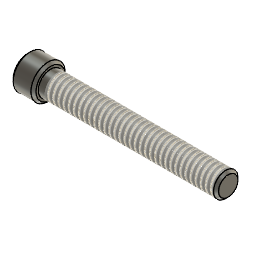
m2 bolt 6mm v2 (Autodesk Fusion 360 design; units mm, degrees)
Autodesk Fusion 360 part; units mm, degrees
sketch "Sketch1" plane through (0, 0, 0) normal (1, 0, 0) x (0, 1, 0)
  circle A0 centre (0, 0) radius 1.35
  line L0 (0, 0.866) -> (-0.75, 0.433)
  line L1 (-0.75, 0.433) -> (-0.75, -0.433)
  line L2 (-0.75, -0.433) -> (0, -0.866)
  line L3 (0, -0.866) -> (0.75, -0.433)
  line L4 (0.75, -0.433) -> (0.75, 0.433)
  line L5 (0.75, 0.433) -> (0, 0.866)
  line L6 (-0.75, -0.433) -> (0.75, 0.433) construction
  line L7 (0.75, -0.433) -> (-0.75, 0.433) construction
  line L8 (0, 0.866) -> (0, -0.866) construction
  line L9 (-0.75, -0.433) -> (0.75, -0.433) construction
  dimension "d1" = 1.5
  dimension "d2" = 2.7
  constraint coincident A0.centre origin
  constraint vertical L1
  constraint parallel L1 L4
  constraint equal L1 L2
  constraint equal L0 L1
  constraint equal L0 L5
  constraint equal L4 L5
  constraint equal L3 L4
  constraint midpoint L7 A0.centre
  constraint equal L6 L7
  constraint equal L7 L8
  measures "d1" distance of L1.end L3.end
  measures "d2" diameter of A0
extrude "Extrude1" add sketch "Sketch1" along normal blind 1.8 contours A0 | L0 L1 L2 L3 L4 L5
extrude "Extrude2" cut sketch "Sketch1" along normal blind 1 contours L0 L1 L2 L3 L4 L5
sketch "Sketch2" plane through (1.8, 0, 0) normal (1, 0, 0) x (0, 1, 0)
  circle A0 centre (0, 0) radius 1.35
  circle A1 centre (0, 0) radius 1
  dimension "d7" = 2
  constraint coincident A0.centre A1.centre
  measures "d7" diameter of A1
extrude "Extrude3" add sketch "Sketch2" along normal blind 14 contours A1
thread "Thread1" "ISO Metric profile 2.0 M2x0.4 M2x0.4 6g" major diameter 1.9335 minor diameter 1.478 pitch 0.4 angle 60 resizes the face on face at (11.1333, 0.995, -0.0996) from (2.3, 0, 0) to (15.8, 0, 0)
chamfer "Chamfer1" distance 0.2 angle 45 3 edges at (15.8, -0.9013, -0.3496) (1.8, -1.2586, -0.4882) (0, -1.2586, -0.4882)
